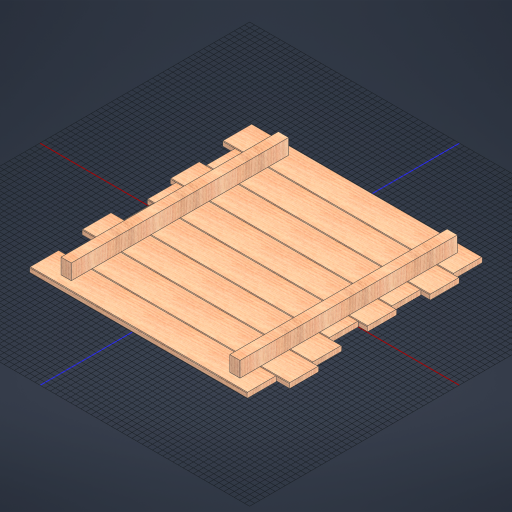
# Autodesk Inventor part: Backboard
Saved by Autodesk Inventor 2023.2 (Build 272271030, 271C)
## iProperties
Created: 2023-02-22
Part Number: Backboard
Material: Holz (Birke)
Document SubType Name: Modeling
Designer: Stefan
Mass: 10942.1 g
Surface Area: 19012.6 cm^2
Volume: 19894.8 cm^3
Density: 0.55 g/cm^3
Appearance: Birke - natur - poliert
Author: Stefan
Autodesk Inventor part; units mm, degrees
ref_plane "YZ Plane" through (0, 0, 0) normal (1, 0, 0) x (0, 1, 0)
ref_plane "XZ Plane" through (0, 0, 0) normal (0, 1, 0) x (-1, 0, 0)
ref_plane "XY Plane" through (0, 0, 0) normal (0, 0, 1) x (1, 0, 0)
sketch "Skizze1" plane through (0, 0, 0) normal (1, 0, 0) x (0, 1, 0)
  line L0 (8, 460) -> (-8, 460)
  line L1 (-10, 458) -> (-10, 347)
  line L2 (-8, 345) -> (8, 345)
  line L3 (10, 347) -> (10, 458)
  line L4 (8, 345) -> (-8, 345)
  line L5 (-10, 343) -> (-10, 232)
  line L6 (-8, 230) -> (8, 230)
  line L7 (10, 232) -> (10, 343)
  line L8 (8, 230) -> (-8, 230)
  line L9 (-10, 228) -> (-10, 117)
  line L10 (-8, 115) -> (8, 115)
  line L11 (10, 117) -> (10, 228)
  line L12 (8, 115) -> (-8, 115)
  line L13 (-10, 113) -> (-10, 2)
  line L14 (-8, 0) -> (8, 0)
  line L15 (10, 2) -> (10, 113)
  line L16 (8, 0) -> (-8, 0)
  line L17 (-10, -2) -> (-10, -113)
  line L18 (-8, -115) -> (8, -115)
  line L19 (10, -113) -> (10, -2)
  line L20 (8, -115) -> (-8, -115)
  line L21 (-10, -117) -> (-10, -228)
  line L22 (-8, -230) -> (8, -230)
  line L23 (10, -228) -> (10, -117)
  line L24 (8, -230) -> (-8, -230)
  line L25 (-10, -232) -> (-10, -343)
  line L26 (-8, -345) -> (8, -345)
  line L27 (10, -343) -> (10, -232)
  line L28 (10, -343) -> (8, -345)
  line L29 (10, -232) -> (8, -230)
  line L30 (10, -228) -> (8, -230)
  line L31 (10, -117) -> (8, -115)
  line L32 (8, -115) -> (10, -113)
  line L33 (10, -2) -> (8, 0)
  line L34 (8, 0) -> (10, 2)
  line L35 (10, 113) -> (8, 115)
  line L36 (8, 115) -> (10, 117)
  line L37 (10, 228) -> (8, 230)
  line L38 (10, 232) -> (8, 230)
  line L39 (10, 343) -> (8, 345)
  line L40 (10, 347) -> (8, 345)
  line L41 (10, 458) -> (8, 460)
  line L42 (-8, -345) -> (-10, -343)
  line L43 (-10, -232) -> (-8, -230)
  line L44 (-10, -228) -> (-8, -230)
  line L45 (-10, -117) -> (-8, -115)
  line L46 (-10, -113) -> (-8, -115)
  line L47 (-10, -2) -> (-8, 0)
  line L48 (-10, 2) -> (-8, 0)
  line L49 (-10, 113) -> (-8, 115)
  line L50 (-10, 117) -> (-8, 115)
  line L51 (-10, 343) -> (-8, 345)
  line L52 (-10, 347) -> (-8, 345)
  line L53 (-8, 460) -> (-10, 458)
  line L54 (8, -345) -> (-8, -345)
  line L55 (-10, -347) -> (-10, -458)
  line L56 (-8, -460) -> (8, -460)
  line L57 (10, -458) -> (10, -347)
  line L58 (8, -345) -> (10, -347)
  line L59 (10, -458) -> (8, -460)
  line L60 (-8, -460) -> (-10, -458)
  line L61 (-10, -347) -> (-8, -345)
  line L62 (-8, 230) -> (-10, 232)
  line L63 (-8, 230) -> (-10, 228)
  point P0 (0, 115)
  point P1 (10, 460)
  point P2 (-10, 345)
  point P3 (-10, 460)
  point P4 (10, 345)
  point P5 (-10, 230)
  point P6 (-10, 345)
  point P7 (10, 230)
  point P8 (-10, 115)
  point P9 (-10, 230)
  point P10 (10, 115)
  point P11 (-10, 0)
  point P12 (-10, 115)
  point P13 (10, 0)
  point P14 (-10, -115)
  point P15 (-10, 0)
  point P16 (10, -115)
  point P17 (-10, -230)
  point P18 (-10, -115)
  point P19 (10, -230)
  point P20 (0, 115)
  point P21 (-10, 230)
  point P22 (-10, 230)
  point P23 (-9, 0)
  point P24 (-9, -115)
  point P25 (-9, -230)
  point P26 (-10, -345)
  point P27 (10, -345)
  point P28 (-10, 0)
  point P29 (-10, 0)
  point P30 (-10, 0)
  point P31 (-10, 115)
  point P32 (-10, 115)
  point P33 (-10, 345)
  point P34 (-10, 345)
  point P35 (-8, -115)
  point P36 (-10, -460)
  point P37 (-10, -345)
  point P38 (10, -460)
  point P39 (0, 0)
  point P40 (0, 0)
  dimension "d0" = 20
  dimension "d1" = 115
  dimension "d30" = 2
  dimension "d31" = 2
  dimension "d32" = 2
  dimension "d33" = 2
  dimension "d34" = 2
  dimension "d35" = 2
  dimension "d36" = 2
  dimension "d37" = 2
  dimension "d38" = 2
  dimension "d39" = 2
  dimension "d40" = 2
  dimension "d41" = 2
  dimension "d42" = 2
  dimension "d43" = 2
  dimension "d44" = 2
  dimension "d45" = 2
  dimension "d46" = 2
  dimension "d47" = 2
  dimension "d48" = 2
  dimension "d49" = 2
  dimension "d50" = 2
  dimension "d51" = 2
  dimension "d52" = 2
  dimension "d53" = 2
  dimension "d54" = 2
  dimension "d55" = 2
  dimension "d56" = 2
  dimension "d57" = 2
  dimension "d58" = 2
  dimension "d59" = 2
  dimension "d60" = 2
  dimension "d61" = 2
  dimension "d62" = 2
  dimension "d63" = 2
  dimension "d64" = 2
  dimension "d65" = 2
  dimension "d66" = 2
  dimension "d67" = 2
  dimension "d68" = 2
  dimension "d69" = 2
  dimension "d70" = 2
  dimension "d71" = 2
  dimension "d72" = 2
  dimension "d73" = 2
  dimension "d74" = 2
  dimension "d75" = 2
  dimension "d76" = 2
  dimension "d77" = 2
  dimension "d78" = 2
  dimension "d79" = 2
  dimension "d80" = 2
  dimension "d81" = 2
  dimension "d90" = 2
  dimension "d91" = 2
  dimension "d92" = 2
  dimension "d93" = 2
  dimension "d94" = 2
  dimension "d95" = 2
  dimension "d96" = 2
  dimension "d97" = 2
  dimension "d102" = 2
  dimension "d103" = 2
  constraints: 128 end point, 81 point on line, 16 parallel, 8 horizontal, 8 perpendicular, 7 collinear, 3 coincident, 2 midpoint
  measures "d0" distance between parallel lines of L1 L3
  measures "d1" distance of point (10, 345) point (10, 460)
  measures "d30" distance of L27.start point (10, -345)
  measures "d31" distance of L26.end point (10, -345)
  measures "d32" distance of L27.end point (10, -230)
  measures "d33" distance of L22.end point (10, -230)
  measures "d34" distance of L23.start point (10, -230)
  measures "d35" distance of L24.start point (10, -230)
  measures "d36" distance of L23.end point (10, -115)
  measures "d37" distance of L18.end point (10, -115)
  measures "d38" distance of L20.start point (10, -115)
  measures "d39" distance of L19.start point (10, -115)
  measures "d40" distance of L19.end point (10, 0)
  measures "d41" distance of L14.end point (10, 0)
  measures "d42" distance of L16.start point (10, 0)
  measures "d43" distance of L15.start point (10, 0)
  measures "d44" distance of L15.end point (10, 115)
  measures "d45" distance of L10.end point (10, 115)
  measures "d46" distance of L12.start point (10, 115)
  measures "d47" distance of L11.start point (10, 115)
  measures "d48" distance of L11.end point (10, 230)
  measures "d49" distance of L6.end point (10, 230)
  measures "d50" distance of L7.start point (10, 230)
  measures "d51" distance of L8.start point (10, 230)
  measures "d52" distance of L7.end point (10, 345)
  measures "d53" distance of L2.end point (10, 345)
  measures "d54" distance of L3.start point (10, 345)
  measures "d55" distance of L4.start point (10, 345)
  measures "d56" distance of L3.end point (10, 460)
  measures "d57" distance of L0.start point (10, 460)
  measures "d58" distance of L26.start point (-10, -345)
  measures "d59" distance of L25.end point (-10, -345)
  measures "d60" distance of L25.start point (-10, -230)
  measures "d61" distance of L22.start point (-10, -230)
  measures "d62" distance of L21.end point (-10, -230)
  measures "d63" distance of L24.end point (-10, -230)
  measures "d64" distance of L21.start point (-10, -115)
  measures "d65" distance of L20.end point (-10, -115)
  measures "d66" distance of L17.end point (-10, -115)
  measures "d67" distance of L18.start point (-10, -115)
  measures "d68" distance of L17.start point (-10, 0)
  measures "d69" distance of L14.start point (-10, 0)
  measures "d70" distance of L13.end point (-10, 0)
  measures "d71" distance of L16.end point (-10, 0)
  measures "d72" distance of L13.start point (-10, 115)
  measures "d73" distance of L10.start point (-10, 115)
  measures "d74" distance of L9.end point (-10, 115)
  measures "d75" distance of L12.end point (-10, 115)
  measures "d76" distance of L5.start point (-10, 345)
  measures "d77" distance of L2.start point (-10, 345)
  measures "d78" distance of L1.end point (-10, 345)
  measures "d79" distance of L4.end point (-10, 345)
  measures "d80" distance of L0.end point (-10, 460)
  measures "d81" distance of L1.start point (-10, 460)
  measures "d90" distance of L54.start point (10, -345)
  measures "d91" distance of L57.end point (10, -345)
  measures "d92" distance of L57.start point (10, -460)
  measures "d93" distance of L56.end point (10, -460)
  measures "d94" distance of L56.start point (-10, -460)
  measures "d95" distance of L55.end point (-10, -460)
  measures "d96" distance of L55.start point (-10, -345)
  measures "d97" distance of L54.end point (-10, -345)
  measures "d102" distance of L6.start point (-10, 230)
  measures "d103" distance of L5.end point (-10, 230)
extrude "Extrusion1" add sketch "Skizze1" along normal blind 450 and the other way blind 400 contours L41 L3 L40 L2 L52 L1 L53 L0
extrude "Extrusion3" add sketch "Skizze1" along normal blind 475 and the other way blind 425 contours L37 L11 L36 L10 L50 L9 L63 L6
extrude "Extrusion2" add sketch "Skizze1" along normal blind 500 and the other way blind 350 contours L39 L7 L38 L6 L62 L5 L51 L2
extrude "Extrusion4" add sketch "Skizze1" along normal blind 425 and the other way blind 375 contours L35 L15 L34 L14 L48 L13 L49 L10
extrude "Extrusion5" add sketch "Skizze1" along normal blind 460 and the other way blind 400 contours L33 L19 L32 L18 L46 L17 L47 L14
extrude "Extrusion6" add sketch "Skizze1" along normal blind 440 and the other way blind 425 contours L31 L23 L30 L22 L44 L21 L45 L18
extrude "Extrusion7" add sketch "Skizze1" along normal blind 475 and the other way blind 400 contours L29 L27 L28 L26 L42 L25 L43 L22
extrude "Extrusion9" add sketch "Skizze1" along normal blind 450 and the other way blind 450 contours L58 L57 L59 L56 L60 L55 L61 L26
sketch "Skizze2" plane through (-400, 10, 458) normal (0, 1, 0) x (1, 0, 0)
  line L0 (747.5, 33) -> (787.5, 33)
  line L1 (787.5, 33) -> (787.5, 883)
  line L2 (787.5, 883) -> (747.5, 883)
  line L3 (747.5, 883) -> (747.5, 33)
  line L4 (87.5, 33) -> (127.5, 33)
  line L5 (127.5, 33) -> (127.5, 883)
  line L6 (127.5, 883) -> (87.5, 883)
  line L7 (87.5, 883) -> (87.5, 33)
  line L8 (87.5, 33) -> (787.5, 33) construction
  line L9 (787.5, 33) -> (787.5, 883) construction
  line L10 (787.5, 883) -> (87.5, 883) construction
  line L11 (87.5, 883) -> (87.5, 33) construction
  line L12 (-25, -2) -> (900, -2) construction
  line L13 (900, -2) -> (900, 918) construction
  line L14 (900, 918) -> (-25, 918) construction
  line L15 (-25, 918) -> (-25, -2) construction
  line L16 (0, -2) -> (850, -2) construction
  line L17 (-25, 230) -> (-25, 341) construction
  line L18 (900, 226) -> (900, 115) construction
  line L19 (0, 803) -> (875, 803) construction
  line L20 (-25, 458) -> (900, 458) construction
  line L21 (0, 803) -> (875, 803) construction
  line L22 (437.5, -2) -> (437.5, 918) construction
  line L23 (-50, 918) -> (850, 918) projected
  point P0 (400, 458)
  point P1 (87.5, 458)
  point P2 (437.5, 33)
  dimension "d82" = 40
  dimension "d83" = 40
  dimension "d84" = 850
  dimension "d85" = 700
  constraints: 34 end point, 7 parallel, 6 horizontal, 5 midpoint, 5 perpendicular, 3 collinear, 3 point on line, 4 other
  measures "d82" distance between parallel lines of L5 L7
  measures "d83" distance between parallel lines of L1 L3
  measures "d84" distance between parallel lines of L10 L8
  measures "d85" distance between parallel lines of L9 L7
extrude "Extrusion8" add sketch "Skizze2" along normal blind 60
equation "\"d31\" = d30"
equation "\"d33\" = d32"
equation "\"d34\" = d32"
equation "\"d35\" = d34"
equation "\"d36\" = d32"
equation "\"d37\" = d36"
equation "\"d38\" = d32"
equation "\"d39\" = d38"
equation "\"d40\" = d32"
equation "\"d41\" = d40"
equation "\"d42\" = d32"
equation "\"d43\" = d42"
equation "\"d44\" = d32"
equation "\"d45\" = d44"
equation "\"d46\" = d32"
equation "\"d47\" = d46"
equation "\"d48\" = d32"
equation "\"d49\" = d48"
equation "\"d50\" = d32"
equation "\"d51\" = d50"
equation "\"d52\" = d32"
equation "\"d53\" = d52"
equation "\"d54\" = d32"
equation "\"d55\" = d54"
equation "\"d56\" = d32"
equation "\"d57\" = d56"
equation "\"d59\" = d58"
equation "\"d60\" = d58"
equation "\"d61\" = d60"
equation "\"d62\" = d58"
equation "\"d63\" = d62"
equation "\"d64\" = d58"
equation "\"d65\" = d64"
equation "\"d66\" = d58"
equation "\"d67\" = d66"
equation "\"d68\" = d58"
equation "\"d69\" = d68"
equation "\"d70\" = d58"
equation "\"d71\" = d70"
equation "\"d72\" = d58"
equation "\"d73\" = d72"
equation "\"d74\" = d58"
equation "\"d75\" = d74"
equation "\"d76\" = d58"
equation "\"d77\" = d76"
equation "\"d78\" = d58"
equation "\"d79\" = d78"
equation "\"d80\" = d58"
equation "\"d81\" = d80"
equation "\"d91\" = d90"
equation "\"d92\" = d90"
equation "\"d93\" = d92"
equation "\"d94\" = d90"
equation "\"d95\" = d94"
equation "\"d96\" = d90"
equation "\"d97\" = d96"
equation "\"d83\" = d82"
